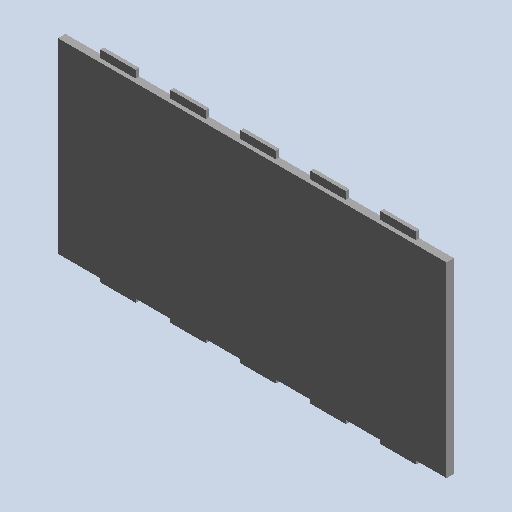
# Autodesk Inventor part: Enclosure_3
Saved by Autodesk Inventor 2026 (Build 300175050, 175E)
## iProperties
Part Number: Enclosure_3
Material: Generic
Document SubType Name: Modeling
Designer: Kartik
Mass: 84.644 g
Surface Area: 457.36 cm^2
Volume: 84.644 cm^3
Density: 1 g/cm^3
Appearance: Default
Author: Kartik
Autodesk Inventor part; units mm, degrees
ref_plane "YZ Plane" through (0, 0, 0) normal (1, 0, 0) x (0, 1, 0)
ref_plane "XZ Plane" through (0, 0, 0) normal (0, 1, 0) x (-1, 0, 0)
ref_plane "XY Plane" through (0, 0, 0) normal (0, 0, 1) x (1, 0, 0)
sketch "Sketch1" plane through (0, 0, 0) normal (0, 0, 1) x (1, 0, 0)
  line L0 (-100.0716, 53.5507) -> (107.9284, 53.5507)
  line L1 (107.9284, 53.5507) -> (107.9284, -46.4493)
  line L2 (107.9284, -46.4493) -> (-100.0716, -46.4493)
  line L3 (-100.0716, -46.4493) -> (-100.0716, 53.5507)
  point P0 (0, 0)
  dimension "d0" = 208
  dimension "d1" = 100
  constraints: 8 end point, 2 parallel, 1 horizontal, 1 perpendicular
  measures "d0" distance of L0.start L0.end
  measures "d1" distance of L0.end L1.end
extrude "Extrusion1" add sketch "Sketch1" along normal blind 4
sketch "Sketch2" plane through (-100.0716, -46.4493, 0) normal (0, -1, 0) x (1, 0, 0)
  line L0 (0, 0) -> (208, 0) projected
  line L1 (20.5, 0) -> (39.5, 0)
  line L2 (39.5, 0) -> (39.5, 1.9)
  line L3 (39.5, 1.9) -> (20.5, 1.9)
  line L4 (20.5, 1.9) -> (20.5, 0)
  line L5 (0, 0) -> (0, 4) projected
  point P0 (100.0716, 0)
  point P1 (20.5, 0.95)
  point P2 (39.5, 0)
  dimension "d4" = 19
  dimension "d5" = 1.9
  dimension "d6" = 20.5
  constraints: 8 end point, 2 parallel, 1 horizontal, 1 midpoint, 1 perpendicular, 1 point on line
  measures "d4" distance of L3.end L2.end
  measures "d5" distance of L2.end L1.end
  measures "d6" distance from line of L5 point (20.5, 0.95)
extrude "Extrusion2" add sketch "Sketch2" along normal blind 4
pattern_linear "Rectangular Pattern1" count 5 spacing 37.5 along (1, 0, 0) count 2 spacing 104 along (0, 1, 0) of "Extrusion2" second direction both ways yes
body "Solid1"
